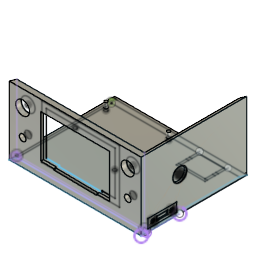
EAP-ControlPanel_v1 (Autodesk Fusion 360 design; units mm, degrees)
Autodesk Fusion 360 part; units mm, degrees
sketch "Sketch1" plane through (0, 0, 0) normal (0, 0, 1) x (1, 0, 0)
  line L0 (-68, -32) -> (-68, 54)
  circle A0 centre (-65, 46) radius 1.45
  circle A1 centre (-65, 18) radius 1.45
  circle A2 centre (-13, 51) radius 1.45
  circle A3 centre (-14, 3) radius 1.45
  line L1 (-70, 59) -> (50, 59)
  line L2 (50, 59) -> (50, -2)
  line L3 (-70, -5) -> (-70, 59)
  line L4 (50, -2) -> (50, -37)
  line L5 (50, -37) -> (-70, -37)
  line L6 (-70, -37) -> (-70, -5)
  line L7 (-68, -32) -> (48, -32)
  line L8 (48, -32) -> (48, 54)
  line L9 (-68, 54) -> (48, 54)
  line L10 (48, -32) -> (50, -37)
  line L11 (-68, -32) -> (-70, -37)
  line L12 (-68, 54) -> (-70, 59)
  line L13 (12, 54) -> (34, 54)
  line L14 (34, 54) -> (34, 37)
  line L15 (34, 37) -> (12, 37)
  line L16 (12, 37) -> (12, 54)
  line L17 (36, 56) -> (36, 35)
  line L18 (36, 35) -> (10, 35)
  line L19 (10, 35) -> (10, 56)
  line L20 (12, 44) -> (10, 44)
  line L21 (10, 47) -> (12, 47)
  line L22 (34, 44) -> (36, 44)
  line L23 (36, 47) -> (34, 47)
  line L24 (12, 54) -> (10, 54)
  line L25 (34, 54) -> (36, 54)
  line L26 (34, 37) -> (36, 37)
  line L27 (12, 37) -> (10, 37)
  line L28 (48, 54) -> (50, 59)
  dimension "d3" = 2.9
  dimension "d5" = 3
  dimension "d6" = 2.9
  dimension "d7" = 3
  dimension "d9" = 2.9
  dimension "d12" = 2.9
  dimension "d17" = 2
  dimension "d26" = 120
  dimension "d27" = 32
  dimension "d28" = 5
  dimension "d29" = 2
  dimension "d30" = 48
  dimension "d32" = 52
  dimension "d33" = 28
  dimension "d34" = 51
  dimension "d36" = 3
  dimension "d37" = 8
  dimension "d75" = 5
  dimension "d76" = 22
  dimension "d77" = 17
  dimension "d78" = 25
  dimension "d81" = 2
  dimension "d82" = 2
  dimension "d83" = 2
  dimension "d84" = 7
  dimension "d85" = 7
  dimension "d86" = 7
  dimension "d87" = 7
  constraint vertical L0
  constraint horizontal L1
  constraint vertical L2
  constraint vertical L3
  constraint vertical L4
  constraint horizontal L5
  constraint vertical L6
  constraint perpendicular L0 L7
  constraint perpendicular L7 L8
  constraint coincident L0.end L9.start
  constraint horizontal L13
  constraint vertical L14
  constraint horizontal L15
  constraint vertical L16
  constraint vertical L17
  constraint horizontal L18
  constraint vertical L19
  constraint coincident L16 L20.start
  constraint coincident L19 L20.end
  constraint perpendicular L19 L20
  constraint coincident L19 L21.start
  constraint coincident L16 L21.end
  constraint perpendicular L16 L21
  constraint coincident L14 L22.start
  constraint coincident L17 L22.end
  constraint perpendicular L17 L22
  constraint coincident L17 L23.start
  constraint coincident L14 L23.end
  constraint perpendicular L14 L23
  constraint coincident L19 L24.end
  constraint perpendicular L19 L24
  constraint coincident L17 L25.end
  constraint perpendicular L17 L25
  constraint coincident L17 L26.end
  constraint perpendicular L17 L26
  constraint coincident L19 L27.end
  constraint perpendicular L19 L27
  constraint collinear L9 L13
  measures "d3" diameter of A0
  measures "d5" distance of L0 A0.centre
  measures "d6" diameter of A1
  measures "d7" distance of L0 A1.centre
  measures "d9" diameter of A2
  measures "d12" diameter of A3
  measures "d17" distance of L0 L3
  measures "d26" distance of L2 L3
  measures "d27" distance of L3.start L5.end
  measures "d28" distance of L5 L7
  measures "d29" distance of L4 L8
  measures "d30" vertical distance of A2.centre A3.centre
  measures "d32" horizontal distance of A0.centre A2.centre
  measures "d33" distance of A0.centre A1.centre
  measures "d34" horizontal distance of A1.centre A3.centre
  measures "d36" distance of A2.centre L9
  measures "d37" distance of A0.centre L9
  measures "d75" distance of L1 L9
  measures "d76" distance of L13.start L13.end
  measures "d77" distance of L13.start L15.end
  measures "d78" distance of A2.centre L16
  measures "d81" distance of L14 L17
  measures "d82" distance of L15 L18
  measures "d83" distance of L16 L19
  measures "d84" distance of L13.start L21.end
  measures "d85" distance of L15 L20.start
  measures "d86" distance of L13 L23.end
  measures "d87" distance of L14.end L22.start
extrude "Extrude1" add sketch "Sketch1" along normal blind 2
extrude "Extrude3" add sketch "Sketch1" along normal blind 7 contours L16 L19 L20 L21 | L14 L17 L22 L23 | L15 L17 L18 L19 L26 L27 | A0 | A1 | A2 | A3
extrude "Extrude4" add sketch "Sketch1" along normal blind 62 contours L5 L7 L10 L11 | L2 L4 L8 L10 L28
sketch "Sketch2" plane through (0, -32, 0) normal (0, 1, 0) x (-1, 0, 0)
  line L0 (68, 62) -> (-48, 62)
  line L1 (-25.25, 56.25) -> (45.25, 56.25)
  line L2 (45.25, 56.25) -> (45.25, 7.75)
  line L3 (45.25, 7.75) -> (-25.25, 7.75)
  line L4 (-25.25, 7.75) -> (-25.25, 56.25)
  line L5 (-21.25, 52.25) -> (41.25, 52.25)
  line L6 (41.25, 52.25) -> (41.25, 13.25)
  line L7 (-21.25, 12.75) -> (-21.25, 52.25)
  line L8 (-21.25, 12.75) -> (-9.5, 12.75)
  line L9 (41.25, 13.25) -> (29.5, 13.25)
  line L10 (-9.5, 11.75) -> (29.5, 12.25)
  line L11 (29.5, 12.25) -> (29.5, 13.25)
  line L12 (-9.5, 12.75) -> (-9.5, 11.75)
  circle A0 centre (-37.75, 47) radius 6
  circle A1 centre (-37.75, 23.5) radius 3
  line L13 (-50, 0) -> (70, 0)
  circle A2 centre (57.75, 47) radius 6.25
  circle A3 centre (57.75, 23.5) radius 3
  line L14 (68, 0) -> (-48, 0)
  line L15 (-48, 2) -> (68, 2)
  line L16 (68, 2) -> (68, 62)
  line L17 (-48, 62) -> (-48, 2)
  dimension "d40" = 70.5
  dimension "d41" = 48.5
  dimension "d43" = 5.75
  dimension "d44" = 62.5
  dimension "d46" = 4
  dimension "d47" = 4
  dimension "d48" = 11.75
  dimension "d49" = 11.75
  dimension "d50" = 1
  dimension "d51" = 1
  dimension "d56" = 12
  dimension "d57" = 6
  dimension "d58" = 12.5
  dimension "d59" = 12.5
  dimension "d60" = 15
  dimension "d61" = 23.5
  dimension "d64" = 6
  dimension "d65" = 12.5
  dimension "d66" = 12.5
  dimension "d67" = 12.5
  dimension "d68" = 23.5
  dimension "d69" = 15
  dimension "d110" = 39.5
  dimension "d111" = 22.75
  constraint horizontal L1
  constraint vertical L2
  constraint horizontal L3
  constraint vertical L4
  constraint horizontal L5
  constraint vertical L6
  constraint vertical L7
  constraint perpendicular L7 L8
  constraint perpendicular L6 L9
  constraint vertical L12
  measures "d40" distance of L1.start L1.end
  measures "d41" distance of L1.start L3.end
  measures "d43" distance of L0 L1
  measures "d44" distance of L5.start L5.end
  measures "d46" distance of L2 L6
  measures "d47" distance of L1 L5
  measures "d48" distance of L7.start L8.end
  measures "d49" distance of L6.end L9.end
  measures "d50" distance of L8.end L10.start
  measures "d51" distance of L9.end L10.end
  measures "d56" diameter of A0
  measures "d57" diameter of A1
  measures "d58" distance of L4 A0.centre
  measures "d59" distance of L4 A1.centre
  measures "d60" distance of L0 A0.centre
  measures "d61" distance of A1.centre L13
  measures "d64" diameter of A3
  measures "d65" diameter of A2
  measures "d66" distance of L2 A2.centre
  measures "d67" distance of L2 A3.centre
  measures "d68" distance of A3.centre L14
  measures "d69" distance of L0 A2.centre
  measures "d110" distance of L5.start L7.start
  measures "d111" distance of L2 L16
extrude "Extrude5" cut sketch "Sketch2" against normal blind 5 contours L5 L6 L7 L8 L9 L10 L11 L12 | A0 | A1 | A2 | A3
extrude "Extrude6" cut sketch "Sketch2" against normal blind 2.5 contours L1 L2 L3 L4
sketch "Sketch4" plane through (50, 0, 0) normal (1, 0, 0) x (0, 1, 0)
  line L0 (-37, 0) -> (59, 0)
  line L1 (59, 0) -> (59, 2)
  line L2 (59, 2) -> (59, 62)
  line L3 (59, 62) -> (-37, 62)
  line L4 (-37, 62) -> (-37, 0)
  circle A0 centre (-2, 31) radius 6.25
  line L5 (-23, 8.5) -> (-13, 8.5)
  line L6 (-13, 8.5) -> (-13, 5)
  line L7 (-13, 5) -> (-23, 5)
  line L8 (-23, 5) -> (-23, 8.5)
  line L9 (-2, 0) -> (-37, 0)
  circle A1 centre (-9.5, 6.75) radius 1.5
  circle A2 centre (-26.5, 6.75) radius 1.5
  line L10 (-31, 10.75) -> (-5, 10.75)
  line L11 (-5, 10.75) -> (-5, 2.75)
  line L12 (-5, 2.75) -> (-31, 2.75)
  line L13 (-31, 2.75) -> (-31, 10.75)
  dimension "d88" = 12.5
  dimension "d89" = 31
  dimension "d90" = 35
  dimension "d93" = 10
  dimension "d94" = 3.5
  dimension "d95" = 5
  dimension "d96" = 14
  dimension "d97" = 3
  dimension "d98" = 3.5
  dimension "d99" = 1.75
  dimension "d100" = 3
  dimension "d101" = 1.75
  dimension "d102" = 3.5
  dimension "d103" = 26
  dimension "d104" = 8
  dimension "d105" = 2.25
  dimension "d106" = 8
  constraint horizontal L5
  constraint vertical L6
  constraint horizontal L7
  constraint vertical L8
  constraint horizontal L10
  constraint vertical L11
  constraint horizontal L12
  constraint vertical L13
  measures "d88" diameter of A0
  measures "d89" distance of L3 A0.centre
  measures "d90" distance of L4 A0.centre
  measures "d93" distance of L5.start L5.end
  measures "d94" distance of L5.start L7.end
  measures "d95" distance of L7 L9
  measures "d96" distance of L4 L8
  measures "d97" diameter of A1
  measures "d98" distance of L6 A1.centre
  measures "d99" distance of L7 A1.centre
  measures "d100" diameter of A2
  measures "d101" distance of L5 A2.centre
  measures "d102" distance of L8 A2.centre
  measures "d103" distance of L10.start L10.end
  measures "d104" distance of L10.start L12.end
  measures "d105" distance of L5 L10
  measures "d106" distance of L6 L11
extrude "Extrude8" cut sketch "Sketch4" against normal blind 2 contours A0 | L5 L6 L7 L8 | A1 | A2
extrude "Extrude9" cut sketch "Sketch4" against normal blind 1 from surface at -1 contours L10 L11 L12 L13
